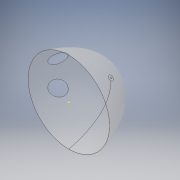
# Autodesk Inventor part: Covering
Saved by Autodesk Inventor 2018 (Build 220112000, 112)
## iProperties
Created: 2019-06-02
Part Number: Covering
Material: Generic
Document SubType Name: Modeling
Designer: dell
Density: 1 g/cm^3
Appearance: Default
Author: dell
Autodesk Inventor part; units mm, degrees
ref_plane "YZ Plane" through (0, 0, 0) normal (1, 0, 0) x (0, 1, 0)
ref_plane "XZ Plane" through (0, 0, 0) normal (0, 1, 0) x (-1, 0, 0)
ref_plane "XY Plane" through (0, 0, 0) normal (0, 0, 1) x (1, 0, 0)
sketch "Sketch1" plane through (0, 0, 0) normal (1, 0, 0) x (0, 1, 0)
  spline S0 degree 2 poles (826.1565, -50) (829.2724, -585.9152) (0, -800) knots 0 0 0 1 1 1
  line L0 (826.1565, -50) -> (826.1565, 0)
  line L1 (826.1565, 0) -> (0, 0)
  line L2 (0, 0) -> (0, -50)
  line L3 (0, -50) -> (0, -800)
  line L4 (-225.8393, 0) -> (1177.5939, 0) projected
  point P0 (676.1565, -450)
  dimension "d0" = 750
  dimension "d1" = 400
  dimension "d2" = 150
  dimension "d3" = 350
  dimension "d4" = 0
  dimension "d5" = 50
  dimension "d6" = 50
  constraints: 8 end point, 1 collinear, 1 perpendicular, 1 vertical, 3 other
  measures "d0" distance of L3.end L2.end
  measures "d1" vertical distance of L0.start point (676.156, -450)
  measures "d2" horizontal distance of L0.start point (676.156, -450)
  measures "d3" vertical distance of point (676.156, -450) L3.end
  measures "d4" horizontal distance of L1.end L2.end
  measures "d5" distance of L1.end L2.end
  measures "d6" vertical distance of L1.end L0.start
revolve "Revolution1" add sketch "Sketch1" angle 360 about axis through (0, -10, 0) along (0, 1, 0)
shell "Shell1" thickness 5 removed faces 2 at (546.8646, 0, 56.3379) at (8.8667, 0, -9.39)
sketch "Sketch2" plane through (0.0278, 821.1565, 0.023) normal (0, -1, 0) x (0.7283119, 0, 0.6852457)
  circle A0 centre (-0.036, 0.0023) radius 15
  dimension "d9" = 30
  constraints: 1 centre point, 1 coincident
  measures "d9" diameter of A0
extrude "Extrusion1" cut sketch "Sketch2" against normal blind 10
sketch "Sketch3" plane through (0, 0, 0) normal (0, -1, 0) x (1, 0, 0)
  point P0 (0, 0)
sketch "Sketch4" plane through (0, 0, 0) normal (1, 0, 0) x (0, 1, 0)
  circle A0 centre (385.7263, 250.411) radius 125
  line L0 (510.7263, 0) -> (0, 0)
  circle A1 centre (385.7263, -250.411) radius 125
  dimension "d12" = 250
  constraints: 2 centre point, 2 end point, 1 horizontal, 1 symmetric about line, 1 other
  measures "d12" diameter of A0
extrude "Extrusion2" cut sketch "Sketch4" against normal through all
body "Solid1"
